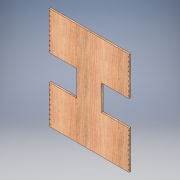
# Autodesk Inventor part: Placeholder Belly Pan
Saved by Autodesk Inventor 2018 (Build 220112000, 112)
## iProperties
Created: 2020-01-18
Part Number: Placeholder Belly Pan
Material: Wood (Birch)
Document SubType Name: Modeling
Designer: maste
Density: 0.55 g/cm^3
Appearance: Birch - Natural Polished
Author: maste
Autodesk Inventor part; units mm, degrees
ref_plane "YZ Plane" through (0, 0, 0) normal (1, 0, 0) x (0, 1, 0)
ref_plane "XZ Plane" through (0, 0, 0) normal (0, 1, 0) x (-1, 0, 0)
ref_plane "XY Plane" through (0, 0, 0) normal (0, 0, 1) x (1, 0, 0)
sketch "Sketch1" plane through (0, 0, 0) normal (0, 0, 1) x (1, 0, 0)
  line L0 (0, 0) -> (476.25, 0)
  line L1 (476.25, 0) -> (476.25, 228.6)
  line L2 (476.25, 228.6) -> (311.15, 228.6)
  line L3 (311.15, 228.6) -> (311.15, 381)
  line L4 (311.15, 381) -> (476.25, 381)
  line L5 (476.25, 381) -> (476.25, 609.6)
  line L6 (476.25, 609.6) -> (0, 609.6)
  line L7 (0, 609.6) -> (0, 381)
  line L8 (0, 381) -> (165.1, 381)
  line L9 (165.1, 381) -> (165.1, 228.6)
  line L10 (165.1, 228.6) -> (0, 228.6)
  line L11 (0, 228.6) -> (0, 0)
  dimension "d0" = 476.25
  dimension "d1" = 228.6
  dimension "d2" = 165.1
  dimension "d3" = 152.4
  dimension "d4" = 228.6
  dimension "d5" = 165.1
  constraints: 24 end point, 8 perpendicular, 7 point on line, 1 horizontal
  measures "d0" distance of L0.start L0.end
  measures "d1" distance of L0.end L1.end
  measures "d2" distance of L1.end L2.end
  measures "d3" distance of L2.end L3.end
  measures "d4" distance of L4.end L5.end
  measures "d5" distance of L7.end L8.end
extrude "Extrusion1" add sketch "Sketch1" along normal blind 9.525
sketch "Sketch2" plane through (0, 0, 9.525) normal (0, 0, 1) x (1, 0, 0)
  line L0 (0, 0) -> (3.175, 0) construction
  line L1 (0, 0) -> (476.25, 0) construction
  line L2 (3.175, 0) -> (3.175, 12.7) construction
  line L3 (3.175, 12.7) -> (3.175, 38.1) construction
  line L4 (3.175, 38.1) -> (3.175, 63.5) construction
  line L5 (3.175, 63.5) -> (3.175, 88.9) construction
  line L6 (3.175, 88.9) -> (3.175, 114.3) construction
  line L7 (3.175, 114.3) -> (3.175, 139.7) construction
  line L8 (3.175, 139.7) -> (3.175, 165.1) construction
  line L9 (3.175, 165.1) -> (3.175, 190.5) construction
  line L10 (3.175, 190.5) -> (3.175, 215.9) construction
  circle A0 centre (3.175, 12.7) radius 2.5797
  circle A1 centre (3.175, 38.1) radius 2.5797
  circle A2 centre (3.175, 63.5) radius 2.5797
  circle A3 centre (3.175, 88.9) radius 2.5797
  circle A4 centre (3.175, 114.3) radius 2.5797
  circle A5 centre (3.175, 139.7) radius 2.5797
  circle A6 centre (3.175, 165.1) radius 2.5797
  circle A7 centre (3.175, 190.5) radius 2.5797
  circle A8 centre (3.175, 215.9) radius 2.5797
  line L11 (238.125, 0) -> (238.125, 609.6) construction
  line L12 (476.25, 609.6) -> (0, 609.6) construction
  line L13 (0, 304.8) -> (476.25, 304.8) construction
  line L14 (473.075, 0) -> (473.075, 12.7) construction
  line L15 (473.075, 12.7) -> (473.075, 38.1) construction
  line L16 (473.075, 38.1) -> (473.075, 63.5) construction
  line L17 (473.075, 63.5) -> (473.075, 88.9) construction
  line L18 (473.075, 88.9) -> (473.075, 114.3) construction
  line L19 (473.075, 114.3) -> (473.075, 139.7) construction
  line L20 (473.075, 139.7) -> (473.075, 165.1) construction
  line L21 (473.075, 165.1) -> (473.075, 190.5) construction
  line L22 (473.075, 190.5) -> (473.075, 215.9) construction
  circle A9 centre (473.075, 12.7) radius 2.5797
  circle A10 centre (473.075, 38.1) radius 2.5797
  circle A11 centre (473.075, 63.5) radius 2.5797
  circle A12 centre (473.075, 88.9) radius 2.5797
  circle A13 centre (473.075, 114.3) radius 2.5797
  circle A14 centre (473.075, 139.7) radius 2.5797
  circle A15 centre (473.075, 165.1) radius 2.5797
  circle A16 centre (473.075, 190.5) radius 2.5797
  circle A17 centre (473.075, 215.9) radius 2.5797
  line L23 (0, 609.6) -> (3.175, 609.6) construction
  line L24 (0, 609.6) -> (476.25, 609.6) construction
  line L25 (3.175, 609.6) -> (3.175, 596.9) construction
  line L26 (3.175, 596.9) -> (3.175, 571.5) construction
  line L27 (3.175, 571.5) -> (3.175, 546.1) construction
  line L28 (3.175, 546.1) -> (3.175, 520.7) construction
  line L29 (3.175, 520.7) -> (3.175, 495.3) construction
  line L30 (3.175, 495.3) -> (3.175, 469.9) construction
  line L31 (3.175, 469.9) -> (3.175, 444.5) construction
  line L32 (3.175, 444.5) -> (3.175, 419.1) construction
  line L33 (3.175, 419.1) -> (3.175, 393.7) construction
  circle A18 centre (3.175, 596.9) radius 2.5797
  circle A19 centre (3.175, 571.5) radius 2.5797
  circle A20 centre (3.175, 546.1) radius 2.5797
  circle A21 centre (3.175, 520.7) radius 2.5797
  circle A22 centre (3.175, 495.3) radius 2.5797
  circle A23 centre (3.175, 469.9) radius 2.5797
  circle A24 centre (3.175, 444.5) radius 2.5797
  circle A25 centre (3.175, 419.1) radius 2.5797
  circle A26 centre (3.175, 393.7) radius 2.5797
  line L34 (473.075, 495.3) -> (473.075, 469.9) construction
  circle A27 centre (473.075, 495.3) radius 2.5797
  line L35 (473.075, 520.7) -> (473.075, 495.3) construction
  line L36 (473.075, 546.1) -> (473.075, 520.7) construction
  line L37 (473.075, 571.5) -> (473.075, 546.1) construction
  line L38 (473.075, 596.9) -> (473.075, 571.5) construction
  circle A28 centre (473.075, 596.9) radius 2.5797
  line L39 (473.075, 609.6) -> (473.075, 596.9) construction
  circle A29 centre (473.075, 520.7) radius 2.5797
  circle A30 centre (473.075, 469.9) radius 2.5797
  circle A31 centre (473.075, 444.5) radius 2.5797
  line L40 (473.075, 444.5) -> (473.075, 419.1) construction
  circle A32 centre (473.075, 419.1) radius 2.5797
  line L41 (473.075, 419.1) -> (473.075, 393.7) construction
  circle A33 centre (473.075, 393.7) radius 2.5797
  circle A34 centre (473.075, 571.5) radius 2.5797
  circle A35 centre (473.075, 546.1) radius 2.5797
  line L42 (473.075, 469.9) -> (473.075, 444.5) construction
  dimension "d8" = 3.175
  dimension "d9" = 12.7
  dimension "d10" = 25.4
  dimension "d11" = 25.4
  dimension "d12" = 25.4
  dimension "d13" = 25.4
  dimension "d14" = 25.4
  dimension "d15" = 25.4
  dimension "d16" = 25.4
  dimension "d17" = 25.4
  dimension "d18" = 5.1594
  constraints: 82 end point, 57 symmetric about line, 36 centre point, 36 coincident, 30 point on line, 2 midpoint, 2 vertical, 1 horizontal, 27 other
  measures "d8" distance of L0.start L0.end
  measures "d9" distance of L0.end L2.end
  measures "d10" distance of L2.end L3.end
  measures "d11" distance of L3.end L4.end
  measures "d12" distance of L4.end L5.end
  measures "d13" distance of L5.end L6.end
  measures "d14" distance of L6.end L7.end
  measures "d15" distance of L7.end L8.end
  measures "d16" distance of L8.end L9.end
  measures "d17" distance of L9.end L10.end
  measures "d18" diameter of A0
extrude "Extrusion2" cut sketch "Sketch2" against normal blind 82.55
body "Solid1"
